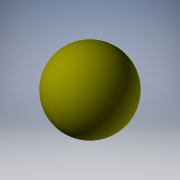
# Autodesk Inventor part: SKF_WBB1-8705-2RS1_ball1
Saved by Autodesk Inventor 2019 (Build 230136000, 136)
## iProperties
Created: 2023-07-31
Part Number: SKF_WBB1-8705-2RS1_ball1
Material: Generic
Catalog Web Link: www.cadenas.de
Description: BB1_001_101_ball1-Deep groove ball bearings
Vendor: SKF
Document SubType Name: Modeling
Designer: psAdmin
Manufacturer: SKF
Mass: 0.000904779 g
Surface Area: 0.0452389 cm^2
Volume: 0.000904779 cm^3
Density: 1 g/cm^3
Appearance: PSOLRGB-175-175-175
Category: PARTsolutions
Company: SKF
Title: SKF_WBB1-8705-2RS1_ball1
Author: Cadenas PARTsolutions
Comments: Deep groove ball bearings
PSOL_IDENT_0: {$CADENAS_DATA/23d-libs/skf/bearings_units_and_housings/ball_bearings/deep_groove_ball_bearings/part
PSOL_IDENT_1: s/bb1_001_101_ball1.prj},202 {VTYP=3D},{NB=SKF_WBB1-8705-2RS1_ball1},{LINA=SKF_WBB1-8705-2RS1_ball1}
PSOL_IDENT_2: ,{NN=BB1_001_101_ball1},{DATE=25.11.2022 05:56:16},{GEOMDATE=21.11.2022 11:35:00},{VERSION=},{LINEID=
PSOL_IDENT_3: 21140},{WBVAR=},{WBNUMERIC=}  {NB=SKF_WBB1-8705-2RS1_ball1},{LINA=SKF_WBB1-8705-2RS1_ball1},{KT=DUMM
PSOL_IDENT_4: Y},{DESIGNATION=WBB1-8705-2RS1},{R12=0.15},{DD=5.000},{D=10.000},{B=4.000},{C=},{CX=},{CXX=},{CA=0.0
PSOL_IDENT_5: 00},{XXVARIANT=},{XXDESIGN=Single row stainless steel},{XXSEALING=Contact seal on both sides},{DESIG
PSOL_IDENT_6: N=dgbb2rs},{DESIGNIR=dgbb2rs},{VARIANT=},{DD1=6.00},{DD2=6},{DD2X=},{DD2A=6.00},{D1=7.80},{D1X=0.00}
PSOL_IDENT_7: ,{D2=8.4},{D2A=8.40},{D3=},{D3X=},{D3A=0.000},{D4=},{HH=0.000},{BB=0.000},{BBX=},{BBA=0.000},{FF=},{
PSOL_IDENT_8: R0MAX=0.000},{R0=0.000},{PITCH=6.90},{DW=1.200},{DDAMIN=5.900},{DDAMAX=5.900},{DDBMIN=0.000},{DDBMAX=
PSOL_IDENT_9: 0.000},{DBMIN=0.000},{DAMAX=8.800},{BBAMIN=0.000},{CAMAX=0.000},{RAMAX=0.150},{LOAD1=0.247},{LOAD2=0
PSOL_IDENT_10: .085},{LOAD3=0.004},{SPEED1=0},{SPEED2=38000},{KR=0.015},{F0=7.600},{Z=8},{II=1},{MASS=0.001},{BEARI
PSOL_IDENT_11: NG=WBB1-8705-2RS1},{RING=},{HELP=1.100},{HELP2=0.800},{DD1ALG=3.000},{YALG=3.000},{PITCH1=6.900},{DW
PSOL_IDENT_12: 1=1.200},{YALG1=3.900},{HALG1=1.100},{SH=3.000},{CU=0.560},{HALG=0.5},{B1=0},{SHIELDHELP=2},{D4A=0.0
PSOL_IDENT_13: 00},{FFA=0.000},{RS1=},{HELP3=0},{SUPPRESS=0}
NB: SKF_WBB1-8705-2RS1_ball1
NN: BB1_001_101_ball1
NT: Deep groove ball bearings
NBSYN: SKF_$DESIGNATION._ball1
LINA: SKF_WBB1-8705-2RS1_ball1
CATALOG: SKF
DESIGNATION: WBB1-8705-2RS1
R12: 0.15
DD: 5
D: 10
B: 4
XXDESIGN: Single row stainless steel
XXSEALING: Contact seal on both sides
DD1: 6
DD2: 6
D1: 7.8
D1X: 0
D2: 8.4
HH: 0
BB: 0
R0MAX: 0
R0: 0
PITCH: 6.9
DW: 1.2
DDAMIN: 5.9
DDAMAX: 5.9
DDBMIN: 0
DDBMAX: 0
DBMIN: 0
DAMAX: 8.8
BBAMIN: 0
CAMAX: 0
RAMAX: 0.15
LOAD1: 0.247
LOAD2: 0.085
LOAD3: 0.004
SPEED1: 0
SPEED2: 38000
KR: 0.015
F0: 7.6
Z: 8
II: 1
MASS: 0.001
BEARING: WBB1-8705-2RS1
HELP3: 0
SUPPRESS: 0
SUPPLIER: SKF
ARTICLENO: SKF_WBB1-8705-2RS1_ball1
BOMINFO: SKF_WBB1-8705-2RS1_ball1
CREATOR: CADENAS GmbH
Autodesk Inventor part; units mm, degrees
sketch "Sketch_6" plane through (0, 0, 0) normal (0, 0, 1) x (1, 0, 0)
  line L0 (2.6, 3.45) -> (1.4, 3.45)
  arc A0 (2.6, 3.45) -> (1.4, 3.45) centre (2, 3.45) ccw
  line L1 (2.6, 3.45) -> (1.4, 3.45)
  constraints: 4 end point, 2 point on circle, 1 centre point
revolve "Revolution1" add sketch "Sketch_6" angle 360 about axis through (2.6, 3.45, 0) along (1, 0, 0)
ref_plane "ball1_XY" through (2, 3.45, 0) normal (1, 0, 0) x (0, 0, -1)
ref_plane "ball1_YZ" through (2, 3.45, 0) normal (0, 0, -1) x (0, 1, 0)
ref_plane "ball1_ZX" through (2, 3.45, 0) normal (0, 1, 0) x (1, 0, 0)
body "Solid1"
